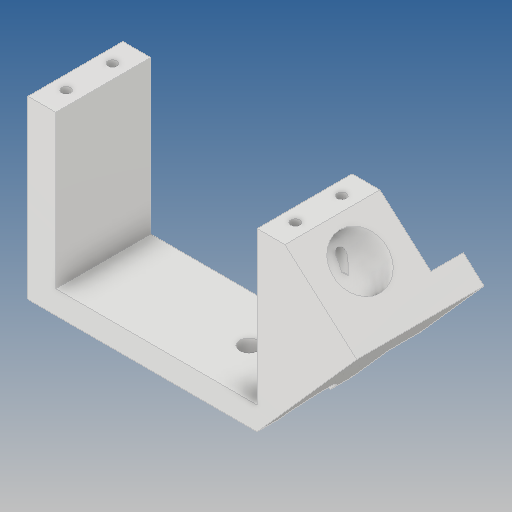
# Autodesk Inventor part: kreplenie3
Saved by Autodesk Inventor 2020 (Build 240168000, 168)
## iProperties
Created: 2019-09-02
Part Number: kreplenie3
Material: Пластик АБС
Document SubType Name: Modeling
Designer: UlyaKZ
Density: 1.06 g/cm^3
Appearance: Гладкий — белый
Author: UlyaKZ
Autodesk Inventor part; units mm, degrees
ref_plane "YZ Plane" through (0, 0, 0) normal (1, 0, 0) x (0, 1, 0)
ref_plane "XZ Plane" through (0, 0, 0) normal (0, 1, 0) x (-1, 0, 0)
ref_plane "XY Plane" through (0, 0, 0) normal (0, 0, 1) x (1, 0, 0)
sketch "Эскиз1" plane through (0, 0, 0) normal (0, 0, 1) x (1, 0, 0)
  line L0 (0, 0) -> (6, 0)
  line L1 (6, 0) -> (6, 38)
  line L2 (6, 38) -> (0, 38)
  line L3 (0, 38) -> (0, 0)
  line L4 (0, 0) -> (49.5, 0)
  line L5 (49.5, 0) -> (49.5, 5)
  line L6 (49.5, 5) -> (0, 5)
  line L7 (0, 5) -> (0, 0)
  line L8 (49.5, 0) -> (55.5, 0) construction
  line L9 (55.5, 0) -> (55.5, 38) construction
  line L10 (55.5, 38) -> (49.5, 38)
  line L11 (49.5, 38) -> (49.5, 0)
  line L12 (49.5, 0) -> (71, 24.2678)
  line L13 (71, 24.2678) -> (55.5, 38)
  dimension "d0" = 5
  dimension "d1" = 6
  dimension "d2" = 43.5
  dimension "d3" = 6
  dimension "d4" = 38
  dimension "d5" = 38
  dimension "d6" = 71
  dimension "d7" = 90
  constraints: 28 end point, 6 parallel, 3 horizontal, 3 perpendicular
  measures "d0" distance between parallel lines of L4 L6
  measures "d1" distance between parallel lines of L3 L1
  measures "d2" distance between parallel lines of L11 L1
  measures "d3" distance between parallel lines of L9 L11
  measures "d4" distance between parallel lines of L8 L10
  measures "d5" distance between parallel lines of L0 L2
  measures "d6" distance from line of L3 L12.end
  measures "d7" angle of L12 L13
extrude "Выдавливание1" add sketch "Эскиз1" along normal blind 20.5
sketch "Эскиз2" plane through (0, 0, 0) normal (0, 0, -1) x (-1, 0, 0)
  line L0 (-49.5, 0) -> (-71, 24.2678) projected
  line L1 (-71, 24.2678) -> (-57.4058, 8.9235)
  line L2 (-57.4058, 8.9235) -> (-52.9148, 12.9023)
  line L3 (-52.9148, 12.9023) -> (-66.509, 28.2466)
  line L4 (-66.509, 28.2466) -> (-71, 24.2678)
  line L5 (-71, 24.2678) -> (-55.5, 38) projected
  line L6 (-58.6417, 14.8426) -> (-55.1603, 10.9129)
  line L7 (-65.273, 22.3276) -> (-68.7545, 26.2572)
  circle A0 centre (-65.273, 22.3276) radius 1
  circle A1 centre (-58.6417, 14.8426) radius 1
  point P0 (0, 0)
  dimension "d10" = 6
  dimension "d11" = 20.5
  dimension "d13" = 2
  dimension "d14" = 2
  dimension "d15" = 8
  constraints: 12 end point, 4 perpendicular, 3 point on line, 2 centre point, 2 coincident, 2 midpoint, 1 collinear
  measures "d10" distance between parallel lines of L0 L3
  measures "d11" distance between parallel lines of L4 L2
  measures "d13" diameter of A0
  measures "d14" diameter of A1
extrude "Выдавливание2" add sketch "Эскиз2" along normal blind 7
sketch "Эскиз3" plane through (49.5, 38, 0) normal (0, 1, 0) x (1, 0, 0)
  circle A0 centre (3, -5.25) radius 1
  circle A1 centre (3, -15.25) radius 1
  circle A2 centre (-46.5, -5.25) radius 1
  circle A3 centre (-46.5, -15.25) radius 1
  line L0 (6, -20.5) -> (0, -20.5) projected
  line L1 (3, -5.25) -> (3, -15.25) construction
  line L2 (6, 0) -> (6, -20.5) projected
  line L3 (-43.5, 0) -> (-49.5, 0) projected
  line L4 (0, 0) -> (0, -20.5) projected
  circle A4 centre (-12, -10.25) radius 2
  point P0 (3, -20.5)
  point P1 (3, -10.25)
  point P2 (6, -10.25)
  point P3 (-46.5, 0)
  point P4 (6, -10.25)
  dimension "d18" = 2
  dimension "d19" = 10
  dimension "d20" = 4
  dimension "d21" = 18
  constraints: 5 centre point, 5 midpoint, 4 horizontal alignment, 4 vertical alignment, 3 equal radius, 2 end point, 1 vertical
  measures "d18" diameter of A2
  measures "d19" distance of L1.end L1.start
  measures "d20" diameter of A4
  measures "d21" distance from line of A4.centre L2
extrude "Выдавливание3" cut sketch "Эскиз3" against normal up to next contours A4
extrude "Выдавливание4" cut sketch "Эскиз3" against normal blind 15 contours A0 | A1 | A2 | A3
sketch "Эскиз4" plane through (55.5, 38, 20.5) normal (0.6631, 0.7485, 0) x (0.7485, -0.6631, 0)
  circle A0 centre (7.958, 10.25) radius 5.75
  line L0 (0, 20.5) -> (0, 0) projected
  line L1 (20.708, 27.5) -> (20.708, 0) projected
  point P0 (-16.3428, 20.5)
  point P1 (0, 10.25)
  dimension "d26" = 7
  dimension "d27" = 11.5
  constraints: 1 centre point, 1 horizontal alignment, 1 midpoint
  measures "d26" distance edge to line of A0 L1
  measures "d27" diameter of A0
extrude "Выдавливание5" cut sketch "Эскиз4" against normal up to next
sketch "Эскиз5" plane through (0, 0, 0) normal (0, -1, 0) x (1, 0, 0)
  circle A0 centre (48.25, 10.25) radius 5.75
  line L0 (49.5, 0) -> (49.5, 20.5) projected
  circle A1 centre (37.5, 10.25) radius 2 projected
  point P0 (0, 0)
  point P1 (49.5, 10.25)
  dimension "d30" = 11.5
  dimension "d31" = 3
  constraints: 1 centre point, 1 horizontal alignment, 1 midpoint
  measures "d30" diameter of A0
extrude "Выдавливание6" cut sketch "Эскиз5" against normal up to next contours A0 L0 | L0 A0
